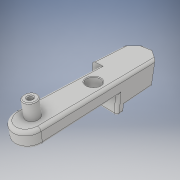
# Autodesk Inventor part: Lift Mount Right
Saved by Autodesk Inventor 2017 (Build 210142000, 142)
## iProperties
Created: 2017-08-10
Part Number: Lift Mount Right
Material: Generic
Document SubType Name: Modeling
Designer: Dale
Density: 1 g/cm^3
Appearance: Default
Author: Dale
## iProperties of the stored document Lift Mount Right_3DPrint.ipt
Created: 2017-08-20
Part Number: Lift Mount Right_3DPrint
Material: Generic
Document SubType Name: Modeling
Designer: Dale
Density: 1 g/cm^3
Appearance: Default
Author: Dale
Autodesk Inventor part; units mm, degrees
ref_plane "YZ Plane" through (0, 0, 0) normal (1, 0, 0) x (0, 1, 0)
ref_plane "XZ Plane" through (0, 0, 0) normal (0, 1, 0) x (-1, 0, 0)
ref_plane "XY Plane" through (0, 0, 0) normal (0, 0, 1) x (1, 0, 0)
sketch "Sketch1" plane through (0, 0, 0) normal (0, 0, 1) x (1, 0, 0)
  line L0 (0, 0) -> (24.5, 0)
  line L1 (24.5, 0) -> (24.5, 19.5)
  line L2 (24.5, 19.5) -> (0, 19.5)
  line L3 (0, 19.5) -> (0, 0)
  dimension "d0" = 19.5
  dimension "d1" = 24.5
  constraints: 8 end point, 2 parallel, 1 horizontal, 1 perpendicular
  measures "d0" distance of L2.end L0.start
  measures "d1" distance of L0.start L0.end
extrude "Extrusion1" add sketch "Sketch1" along normal blind 36.5
sketch "Sketch12" plane through (0, 0, 0) normal (0, -1, 0) x (1, 0, 0)
  line L0 (24.5, 0) -> (24.5, 36.5) projected
  line L1 (0, 0) -> (0, 36.5) projected
  line L2 (24.5, 0) -> (24.5, 36.5) projected
  line L3 (24.5, 9.75) -> (24.5, 0)
  line L4 (0, 0) -> (24.5, 0) projected
  line L5 (14.75, 0) -> (24.5, 9.75)
  line L6 (0, 0) -> (0, 36.5) projected
  line L7 (0, 9.75) -> (9.75, 0)
  line L8 (9.75, 0) -> (0, 0)
  line L9 (0, 0) -> (0, 9.75)
  dimension "d75" = 5
  dimension "d76" = 45
  dimension "d77" = 45
  dimension "d79" = 9.75
  constraints: 10 end point, 3 point on line, 2 perpendicular, 1 collinear
  measures "d75" distance of L7.end L5.start
  measures "d76" angle of L4 L5
  measures "d77" angle of L4 L7
  measures "d79" distance of L1.start L7.end
extrude "Extrusion10" cut sketch "Sketch12" against normal through all
sketch "Sketch2" plane through (0, 0, 36.5) normal (0, 0, 1) x (1, 0, 0)
  line L0 (6.5, 9.5) -> (24.5, 9.5)
  line L1 (24.5, 9.5) -> (24.5, 19.5)
  line L2 (24.5, 19.5) -> (6.5, 19.5)
  line L3 (6.5, 19.5) -> (6.5, 9.5)
  line L4 (0, 0) -> (24.5, 0) projected
  line L5 (24.5, 0) -> (24.5, 19.5) projected
  line L6 (24.5, 19.5) -> (0, 19.5) projected
  dimension "d4" = 10
  dimension "d6" = 18
  constraints: 8 end point, 2 collinear, 2 parallel, 1 horizontal, 1 perpendicular
  measures "d4" distance of L2.end L0.start
  measures "d6" distance of L1.end L2.end
extrude "Extrusion2" add sketch "Sketch2" along normal blind 65
sketch "Sketch3" plane through (6.5, 9.5, 36.5) normal (0, -1, 0) x (1, 0, 0)
  circle A0 centre (9, 15) radius 4.95
  line L0 (18, 0) -> (18, 65) projected
  line L1 (18, 0) -> (0, 0) projected
  line L2 (0, 65) -> (18, 65) projected
  point P0 (-6.5, -36.5)
  point P1 (9, 65)
  dimension "d9" = 9.9
  dimension "d11" = 15
  constraints: 1 centre point, 1 midpoint, 1 vertical alignment
  measures "d9" diameter of A0
  measures "d11" distance from line of L1 A0.centre
extrude "Extrusion3" cut sketch "Sketch3" against normal up to next
sketch "Sketch9" plane through (6.5, 19.5, 35) normal (0, 1, 0) x (1, 0, 0)
  circle A0 centre (9, -55) radius 4
  line L0 (18, -66.5) -> (0, -66.5) projected
  line L1 (18, 0) -> (0, 0) projected
  point P0 (-6.5, 35)
  point P1 (9, -66.5)
  dimension "d42" = 8
  dimension "d43" = 55
  constraints: 1 centre point, 1 midpoint, 1 vertical alignment
  measures "d42" diameter of A0
  measures "d43" distance from line of A0.centre L1
extrude "Extrusion9" add sketch "Sketch9" along normal blind 10
sketch "Sketch14" plane through (0, 0, 36.5) normal (0, 0, 1) x (1, 0, 0)
  line L0 (24.5, 9.5) -> (6.5, 9.5) projected
  line L1 (24.5, 9.5) -> (6.5, 9.5)
  line L2 (6.5, 9.5) -> (6.5, -5)
  line L3 (6.5, -5) -> (24.5, -5)
  line L4 (24.5, -5) -> (24.5, 9.5)
  line L5 (6.5, 9.5) -> (6.5, 19.5) projected
  line L6 (0, 0) -> (24.5, 0) projected
  dimension "d89" = 5
  constraints: 8 end point, 2 parallel, 1 collinear, 1 horizontal, 1 perpendicular
  measures "d89" distance between parallel lines of L3 L6
extrude "Extrusion11" add sketch "Sketch14" along normal blind 5
fillet "Fillet3" radius 9 2 edges at (24.5, 14.5, 101.5) (6.5, 14.5, 101.5)
fillet "Fillet1" radius 2 15 edges at (12.25, 0, 0) (24.5, 0, 23.125) (0, 0, 23.125) (0, 19.5, 23.125) (12.25, 19.5, 0) (21.864, 19.5, 98.864) (9.136, 19.5, 98.864) (6.5, 19.5, 64.5001) (21.864, 9.5, 98.864) (15.5, 9.5, 101.5) (24.5, 9.5, 67.0001) (6.5, 9.5, 67.0001) (24.5, 2.25, 41.5) (24.5, -5, 39) (15.5, -5, 41.5)
fillet "Fillet5" radius 0.5 2 edges at (10.55, 9.5, 51.5) (10.55, 19.5, 51.5)
fillet "Fillet6" radius 0.5 1 edges at (11.5, 29.5, 90)
sketch "Sketch10" plane through (15.5, 29.5, 90) normal (0, 1, 0) x (1, 0, 0)
  point P0 (-15.5, 90)
  point P1 (0, 0)
hole "Upper Arm Cap Hole" at (15.5, 29.5, 90) direction (0, -1, 0) diameter 3 depth 8 tip angle 118 countersink diameter 4 countersink angle 90
sketch "Sketch13" plane through (0, 0, 0) normal (0, 0, -1) x (-1, 0, 0)
  line L0 (-14.75, 17.5) -> (-14.75, 2) projected
  line L1 (-9.75, 2) -> (-14.75, 2) projected
  point P0 (0, 0)
  point P1 (-12.25, 9.75)
  point P2 (-14.75, 9.75)
  point P3 (-12.25, 2)
  constraints: 2 midpoint, 1 horizontal alignment, 1 vertical alignment
hole "Hole3" at (12.25, 9.75, 0) direction (0, 0, 1) diameter 3 depth 10 tip angle 118 countersink diameter 4 countersink angle 90
body "Solid1"
